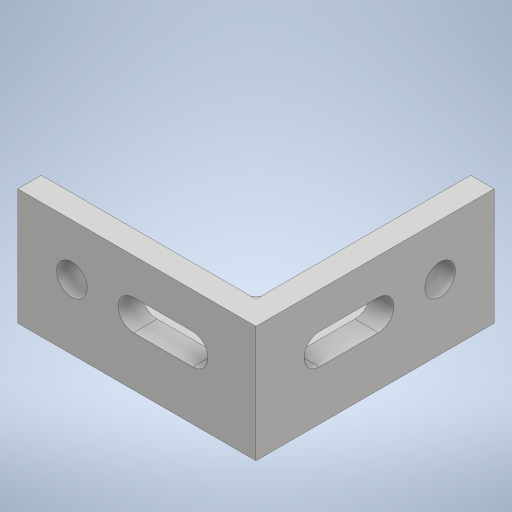
# Autodesk Inventor part: escuadra grande
Saved by Autodesk Inventor 2024.2 (Build 282272000, 272)
## iProperties
Created: 2025-07-02
Part Number: escuadra grande
Material: Genérico
Document SubType Name: Modeling
Designer: jd.castellanosq
Density: 1 g/cm^3
Appearance: Valor por defecto
Author: jd.castellanosq
Autodesk Inventor part; units mm, degrees
ref_plane "YZ Plane" through (0, 0, 0) normal (1, 0, 0) x (0, 1, 0)
ref_plane "XZ Plane" through (0, 0, 0) normal (0, 1, 0) x (-1, 0, 0)
ref_plane "XY Plane" through (0, 0, 0) normal (0, 0, 1) x (1, 0, 0)
sketch "Boceto1" plane through (0, 0, 0) normal (0, 0, 1) x (1, 0, 0)
  line L0 (0, 0) -> (88, 0)
  line L1 (88, 0) -> (88, 88)
  line L2 (88, 88) -> (79.3, 88)
  line L3 (79.3, 88) -> (79.3, 8.7)
  line L4 (79.3, 8.7) -> (0, 8.7)
  line L5 (0, 8.7) -> (0, 0)
  dimension "d0" = 8.7
  dimension "d1" = 8.7
  dimension "d2" = 88
  dimension "d3" = 88
  constraints: 12 end point, 5 perpendicular, 1 horizontal
  measures "d0" distance between parallel lines of L4 L0
  measures "d1" distance between parallel lines of L1 L3
  measures "d2" distance of L0.start L0.end
  measures "d3" distance of L0.end L1.end
extrude "Extrusión1" add sketch "Boceto1" along normal blind 43
sketch "Boceto2" plane through (0, 0, 0) normal (0, 0, -1) x (-1, 0, 0)
  line L0 (-88, 88) -> (-79.3, 88) projected
  line L1 (-79.3, 88) -> (-71.8, 88)
  line L2 (-71.8, 88) -> (-71.8, 79)
  line L3 (-71.8, 79) -> (-9, 16.2)
  line L4 (-9, 16.2) -> (0, 16.2)
  line L5 (-79.3, 88) -> (-79.3, 8.7) projected
  line L6 (-79.3, 8.7) -> (0, 8.7) projected
  line L7 (0, 8.7) -> (0, 16.2)
  point P0 (0, 0)
  dimension "d6" = 7.5
  dimension "d7" = 7.5
  dimension "d8" = 9
  dimension "d9" = 9
  constraints: 10 end point, 1 horizontal, 1 parallel, 1 perpendicular, 1 vertical
  measures "d6" distance between parallel lines of L5 L2
  measures "d7" distance between parallel lines of L6 L4
  measures "d8" distance of L1.end L2.end
  measures "d9" distance of L3.end L4.end
extrude "Extrusión2" add sketch "Boceto2" against normal blind 5
sketch "Boceto3" plane through (79.3, 8.7, 43) normal (-1, 0, 0) x (0, 0, 1)
  line L0 (-19, 36.55) -> (-19, 14.65) construction
  line L1 (-24.65, 36.55) -> (-24.65, 14.65)
  line L2 (-13.35, 14.65) -> (-13.35, 36.55)
  arc A0 (-13.35, 36.55) -> (-24.65, 36.55) centre (-19, 36.55) ccw
  arc A1 (-24.65, 14.65) -> (-13.35, 14.65) centre (-19, 14.65) ccw
  circle A2 centre (-19, 59.3) radius 5.65
  line L3 (-38, 79.3) -> (0, 79.3) projected
  line L4 (-38, 0) -> (0, 0) projected
  point P0 (-43, -8.7)
  point P1 (-19, 25.6)
  point P2 (-19, 79.3)
  point P3 (-19, 9)
  point P4 (-19, 42.2)
  dimension "d12" = 11.3
  dimension "d13" = 20
  dimension "d14" = 11.3
  dimension "d15" = 33.2
  dimension "d16" = 9
  constraints: 8 end point, 6 point on circle, 4 tangent, 3 centre point, 2 midpoint, 2 vertical alignment, 1 parallel, 1 vertical
  measures "d12" diameter of A2
  measures "d13" distance from line of L3 A2.centre
  measures "d14" distance between parallel lines of L2 L1
  measures "d15" distance of point (-19, 9) point (-19, 42.2)
  measures "d16" distance from line of L4 point (-19, 9)
extrude "Extrusión3" cut sketch "Boceto3" against normal through all
sketch "Boceto4" plane through (0, 8.7, 43) normal (0, 1, 0) x (1, 0, 0)
  circle A0 centre (20, 19) radius 5.65
  line L0 (64.65, 19) -> (42.75, 19) construction
  line L1 (64.65, 24.65) -> (42.75, 24.65)
  line L2 (42.75, 13.35) -> (64.65, 13.35)
  arc A1 (64.65, 13.35) -> (64.65, 24.65) centre (64.65, 19) ccw
  arc A2 (42.75, 24.65) -> (42.75, 13.35) centre (42.75, 19) ccw
  line L3 (0, 38) -> (0, 0) projected
  line L4 (79.3, 38) -> (79.3, 0) projected
  point P0 (0, 43)
  point P1 (53.7, 19)
  point P2 (0, 19)
  point P3 (70.3, 19)
  point P4 (37.1, 19)
  dimension "d19" = 11.3
  dimension "d20" = 11.3
  dimension "d21" = 9
  dimension "d22" = 33.2
  dimension "d23" = 20
  constraints: 8 end point, 6 point on circle, 4 tangent, 3 centre point, 2 horizontal alignment, 2 midpoint, 1 horizontal, 1 parallel
  measures "d19" diameter of A0
  measures "d20" distance between parallel lines of L2 L1
  measures "d21" distance from line of L4 point (70.3, 19)
  measures "d22" distance of point (37.1, 19) point (70.3, 19)
  measures "d23" distance from line of L3 A0.centre
extrude "Extrusión4" cut sketch "Boceto4" against normal through all
equation "\"d1\" = d0"
equation "\"d3\" = d2"
equation "\"d7\" = d6"
equation "\"d14\" = d12"
equation "\"d20\" = d19"
